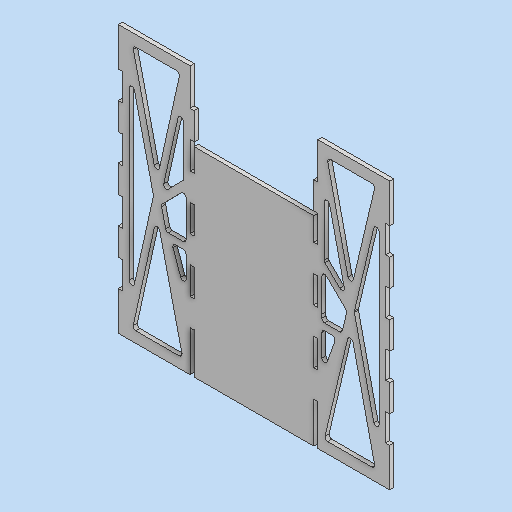
# Autodesk Inventor part: back plate
Saved by Autodesk Inventor 2026 (Build 300175000, 175)
## iProperties
Created: 2026-02-11
Part Number: back plate
Material: Generic
Document SubType Name: Modeling
Designer: mones
Density: 1 g/cm^3
Appearance: Default
Author: mones
Autodesk Inventor part; units mm, degrees
ref_plane "YZ Plane" through (0, 0, 0) normal (1, 0, 0) x (0, 1, 0)
ref_plane "XZ Plane" through (0, 0, 0) normal (0, 1, 0) x (-1, 0, 0)
ref_plane "XY Plane" through (0, 0, 0) normal (0, 0, 1) x (1, 0, 0)
sketch "Sketch1" plane through (0, 0, 0) normal (0, 0, 1) x (1, 0, 0)
  line L0 (-100, 98.5) -> (100, -98.5) construction
  line L1 (100, 98.5) -> (-100, -98.5) construction
  line L2 (-100, 98.5) -> (-100, 70)
  line L3 (-100, 50) -> (-100, 30)
  line L4 (-100, 10) -> (-100, -10)
  line L5 (-100, -30) -> (-100, -50)
  line L6 (-100, -70) -> (-100, -98.5)
  line L7 (-100, 98.5) -> (-100, 95.5)
  line L8 (-100, 98.5) -> (-100, 95.5)
  line L9 (-100, 98.5) -> (-97, 98.5)
  line L10 (-100, -70) -> (-97, -70)
  line L11 (-100, -50) -> (-97, -50)
  line L12 (-100, -30) -> (-97, -30)
  line L13 (-100, -10) -> (-97, -10)
  line L14 (-100, 10) -> (-97, 10)
  line L15 (-100, 30) -> (-97, 30)
  line L16 (-100, 50) -> (-97, 50)
  line L17 (-100, 70) -> (-97, 70)
  line L18 (-100, -98.5) -> (-100, -70)
  line L19 (-100, -50) -> (-100, -30)
  line L20 (-100, -10) -> (-100, 10)
  line L21 (-100, 30) -> (-100, 50)
  line L22 (-100, 70) -> (-100, 98.5)
  line L23 (100, 98.5) -> (97, 98.5)
  line L24 (100, -98.5) -> (100, -70)
  line L25 (100, -50) -> (100, -30)
  line L26 (100, -10) -> (100, 10)
  line L27 (100, 30) -> (100, 50)
  line L28 (100, 70) -> (97, 70)
  line L29 (100, 50) -> (97, 50)
  line L30 (100, 30) -> (97, 30)
  line L31 (100, 10) -> (97, 10)
  line L32 (100, -10) -> (97, -10)
  line L33 (100, -30) -> (97, -30)
  line L34 (100, -50) -> (97, -50)
  line L35 (100, -70) -> (97, -70)
  line L36 (100, -70) -> (100, -98.5)
  line L37 (100, -30) -> (100, -50)
  line L38 (100, 10) -> (100, -10)
  line L39 (100, 98.5) -> (100, 70)
  line L40 (100, 50) -> (100, 30)
  line L41 (-97, -98.5) -> (-47, -98.5)
  line L42 (-47, -98.5) -> (-47, -68.5)
  line L43 (-47, -48.5) -> (-47, -28.5)
  line L44 (-47, -8.5) -> (-47, 11.5)
  line L45 (-47, 31.5) -> (-47, 51.5)
  line L46 (-47, 71.5) -> (-47, 98.5)
  line L47 (-47, 71.5) -> (-44, 71.5)
  line L48 (-47, 51.5) -> (-44, 51.5)
  line L49 (-47, 31.5) -> (-44, 31.5)
  line L50 (-47, 11.5) -> (-44, 11.5)
  line L51 (-47, -8.5) -> (-44, -8.5)
  line L52 (-47, -28.5) -> (-44, -28.5)
  line L53 (-47, -68.5) -> (-44, -68.5)
  line L54 (-47, -98.5) -> (-100, -98.5)
  line L55 (-44, -28.5) -> (-44, -48.5)
  line L56 (-44, -48.5) -> (-47, -48.5)
  line L57 (-44, -98.5) -> (-44, -68.5)
  line L58 (-47, -68.5) -> (-47, -98.5)
  line L59 (-44, -48.5) -> (-44, -28.5)
  line L60 (-47, -28.5) -> (-47, -48.5)
  line L61 (-44, -8.5) -> (-44, 11.5)
  line L62 (-47, 11.5) -> (-47, -8.5)
  line L63 (-44, 31.5) -> (-44, 48.5)
  line L64 (-47, 98.5) -> (-47, 71.5)
  line L65 (-47, 51.5) -> (-47, 31.5)
  line L66 (-100, 98.5) -> (-47, 98.5)
  line L67 (100, -98.5) -> (47, -98.5)
  line L68 (47, -98.5) -> (47, -68.5)
  line L69 (47, -48.5) -> (47, -28.5)
  line L70 (47, -8.5) -> (47, 11.5)
  line L71 (47, 31.5) -> (47, 51.5)
  line L72 (47, 71.5) -> (47, 98.5)
  line L73 (47, 71.5) -> (44, 71.5)
  line L74 (47, 51.5) -> (44, 51.5)
  line L75 (47, 31.5) -> (44, 31.5)
  line L76 (47, 11.5) -> (44, 11.5)
  line L77 (47, -8.5) -> (44, -8.5)
  line L78 (47, -28.5) -> (44, -28.5)
  line L79 (47, -68.5) -> (44, -68.5)
  line L80 (44, -28.5) -> (44, -48.5)
  line L81 (44, -48.5) -> (47, -48.5)
  line L82 (44, -98.5) -> (44, -68.5)
  line L83 (47, -68.5) -> (47, -98.5)
  line L84 (44, -48.5) -> (44, -28.5)
  line L85 (47, -28.5) -> (47, -48.5)
  line L86 (44, -8.5) -> (44, 11.5)
  line L87 (47, 11.5) -> (47, -8.5)
  line L88 (44, 31.5) -> (44, 48.5)
  line L89 (47, 98.5) -> (47, 71.5)
  line L90 (47, 51.5) -> (47, 31.5)
  line L91 (100, -98.5) -> (47, -98.5)
  line L92 (44, -98.5) -> (-44, -98.5)
  line L93 (47, 98.5) -> (97, 98.5)
  line L94 (47, 98.5) -> (100, 98.5)
  line L95 (-97, 98.5) -> (-47, 98.5)
  line L96 (-97, 70) -> (-97, 50)
  line L97 (-97, 30) -> (-97, 10)
  line L98 (-97, -10) -> (-97, -30)
  line L99 (-97, -50) -> (-97, -70)
  line L100 (97, -50) -> (97, -70)
  line L101 (97, -10) -> (97, -30)
  line L102 (97, 30) -> (97, 10)
  line L103 (97, 70) -> (97, 50)
  line L104 (44, 71.5) -> (44, 51.5)
  line L105 (44, 48.5) -> (-44, 48.5)
  line L106 (-44, 71.5) -> (-44, 51.5)
  point P0 (0, 0)
  constraints: 214 end point, 100 perpendicular, 37 parallel, 7 collinear, 4 point on line, 3 horizontal, 2 midpoint
extrude "Extrusion1" add sketch "Sketch1" along normal blind 3
sketch "Sketch2" plane through (0, 0, 3) normal (0, 0, 1) x (1, 0, 0)
  line L0 (-100, -70) -> (-100, -98.5) projected
  line L1 (-100, -98.5) -> (-47, -98.5) projected
  line L2 (-47, -98.5) -> (-47, -68.5) projected
  line L3 (-47, -68.5) -> (-44, -68.5) projected
  line L4 (-44, -68.5) -> (-44, -98.5) projected
  line L5 (-44, -98.5) -> (44, -98.5) projected
  line L6 (44, -98.5) -> (44, -68.5) projected
  line L7 (44, -68.5) -> (47, -68.5) projected
  line L8 (47, -68.5) -> (47, -98.5) projected
  line L9 (47, -98.5) -> (100, -98.5) projected
  line L10 (100, -98.5) -> (100, -70) projected
  line L11 (100, -70) -> (97, -70) projected
  line L12 (97, -70) -> (97, -50) projected
  line L13 (97, -50) -> (100, -50) projected
  line L14 (100, -50) -> (100, -30) projected
  line L15 (100, -30) -> (97, -30) projected
  line L16 (97, -30) -> (97, -10) projected
  line L17 (97, -10) -> (100, -10) projected
  line L18 (100, -10) -> (100, 10) projected
  line L19 (100, 10) -> (97, 10) projected
  line L20 (97, 10) -> (97, 30) projected
  line L21 (97, 30) -> (100, 30) projected
  line L22 (100, 30) -> (100, 50) projected
  line L23 (100, 50) -> (97, 50) projected
  line L24 (97, 50) -> (97, 70) projected
  line L25 (97, 70) -> (100, 70) projected
  line L26 (100, 70) -> (100, 98.5) projected
  line L27 (100, 98.5) -> (47, 98.5) projected
  line L28 (47, 98.5) -> (47, 71.5) projected
  line L29 (47, 71.5) -> (44, 71.5) projected
  line L30 (44, 71.5) -> (44, 51.5) projected
  line L31 (44, 51.5) -> (47, 51.5) projected
  line L32 (47, 51.5) -> (47, 31.5) projected
  line L33 (47, 31.5) -> (44, 31.5) projected
  line L34 (44, 31.5) -> (44, 48.5) projected
  line L35 (44, 48.5) -> (-44, 48.5) projected
  line L36 (-44, 48.5) -> (-44, 31.5) projected
  line L37 (-44, 31.5) -> (-47, 31.5) projected
  line L38 (-47, 31.5) -> (-47, 51.5) projected
  line L39 (-47, 51.5) -> (-44, 51.5) projected
  line L40 (-44, 51.5) -> (-44, 71.5) projected
  line L41 (-44, 71.5) -> (-47, 71.5) projected
  line L42 (-47, 71.5) -> (-47, 98.5) projected
  line L43 (-47, 98.5) -> (-100, 98.5) projected
  line L44 (-100, 98.5) -> (-100, 70) projected
  line L45 (-100, 70) -> (-97, 70) projected
  line L46 (-97, 70) -> (-97, 50) projected
  line L47 (-97, 50) -> (-100, 50) projected
  line L48 (-100, 50) -> (-100, 30) projected
  line L49 (-100, 30) -> (-97, 30) projected
  line L50 (-97, 30) -> (-97, 10) projected
  line L51 (-97, 10) -> (-100, 10) projected
  line L52 (-100, 10) -> (-100, -10) projected
  line L53 (-100, -10) -> (-97, -10) projected
  line L54 (-97, -10) -> (-97, -30) projected
  line L55 (-97, -30) -> (-100, -30) projected
  line L56 (-100, -30) -> (-100, -50) projected
  line L57 (-100, -50) -> (-97, -50) projected
  line L58 (-97, -50) -> (-97, -70) projected
  line L59 (-97, -70) -> (-100, -70) projected
  line L60 (-47, 11.5) -> (-44, 11.5) projected
  line L61 (-44, 11.5) -> (-44, -8.5) projected
  line L62 (-44, -8.5) -> (-47, -8.5) projected
  line L63 (-47, -8.5) -> (-47, 11.5) projected
  line L64 (47, -8.5) -> (44, -8.5) projected
  line L65 (44, -8.5) -> (44, 11.5) projected
  line L66 (44, 11.5) -> (47, 11.5) projected
  line L67 (47, 11.5) -> (47, -8.5) projected
  line L68 (44, -28.5) -> (47, -28.5) projected
  line L69 (47, -28.5) -> (47, -48.5) projected
  line L70 (47, -48.5) -> (44, -48.5) projected
  line L71 (44, -48.5) -> (44, -28.5) projected
  line L72 (-47, -28.5) -> (-44, -28.5) projected
  line L73 (-44, -28.5) -> (-44, -48.5) projected
  line L74 (-44, -48.5) -> (-47, -48.5) projected
  line L75 (-47, -48.5) -> (-47, -28.5) projected
  line L76 (51.6706, 24.0323) -> (51.7144, 61.2135)
  line L77 (50.0544, 13.1843) -> (49.999, -11.4223)
  line L78 (50, -39.3414) -> (50, -23)
  line L79 (-50.0184, -23.0136) -> (-50.0321, -39.1948)
  line L80 (-50, 13.0588) -> (-50, -11.5)
  line L81 (47, 31.5) -> (44, 31.5)
  line L82 (-47, 90.5) -> (-46.8853, 90.4938)
  line L83 (86.8574, 90.5429) -> (56.2449, 90.5429)
  line L84 (-56.9156, 90.4938) -> (-86.863, 90.4938)
  line L85 (-100, 98.5) -> (-52, 98.5)
  line L86 (52, 98.5) -> (97, 98.5)
  line L87 (60.4802, 84.2685) -> (35.0176, 85.6502)
  line L88 (100, 98.5) -> (100, 70)
  line L89 (100, -30) -> (100, -50)
  line L90 (54.2742, -90.4539) -> (86.9163, -90.4539)
  line L91 (47, -98.5) -> (44, -98.5)
  line L92 (-44, -98.5) -> (-100, -98.5)
  line L93 (-86.9859, -90.4916) -> (-54.9903, -90.4916)
  line L94 (-100, -98.5) -> (-100, -70)
  line L95 (-100, -50) -> (-100, -30)
  line L96 (-100, -10) -> (-100, 10)
  line L97 (-100, 30) -> (-100, 98.5)
  line L98 (-51.9599, 60.5849) -> (-52, 26.5)
  line L99 (-95.4597, 94.3495) -> (-47.5647, -89.9349) construction
  line L100 (-52.3399, -91.0567) -> (-90.4937, 95.4882) construction
  line L101 (-93.4655, -85.5459) -> (-49.5589, 89.9605) construction
  line L102 (-54.9518, 88.1154) -> (-88.6187, -86.617) construction
  line L103 (88.5429, -86.5805) -> (54.3944, 91.0824) construction
  line L104 (49.5589, 89.9605) -> (93.4655, -85.5459) construction
  line L105 (48.5891, -85.5203) -> (94.4353, 89.9349) construction
  line L106 (89.4893, 90.9575) -> (52.6562, -86.6086) construction
  line L107 (54.2942, 88.1013) -> (69.2477, 22.0411)
  line L108 (73.9725, 1.696) -> (88.2518, -61.386)
  line L109 (73.1444, 22.0213) -> (88.8035, 88.0816)
  line L110 (88.2563, 62.8381) -> (73.977, 2.5988)
  line L111 (66.5133, 13.728) -> (55.665, 61.6527)
  line L112 (69.0254, -17.5526) -> (52.6562, -86.6086)
  line L113 (88.867, -88.0123) -> (72.9221, -17.5723)
  line L114 (52.6562, -86.6086) -> (52.3281, -87.9926)
  line L115 (92.2024, -60.9445) -> (92.2024, 62.3768)
  line L116 (-73.4539, 22.0984) -> (-88.8109, 88.0401)
  line L117 (-69.5535, 22.1188) -> (-55.2275, 86.6843)
  line L118 (-88.0475, -61.101) -> (-74.1053, 1.7347)
  line L119 (-73.3278, -17.7028) -> (-88.9385, -88.0583)
  line L120 (-88.0521, 62.4881) -> (-74.1099, 2.6215)
  line L121 (-69.4274, -17.6824) -> (-53.0424, -88.0379)
  line L122 (-92, 62.0345) -> (-92, -60.6678)
  line L123 (47.643, -57.6667) -> (66.4978, -19.3333) construction
  line L124 (61.7837, -17.6667) -> (52.357, -59.3333) construction
  line L125 (51.999, -16) -> (63.152, -16)
  line L126 (49.999, -16) -> (64.1404, -20.9995) construction
  line L127 (64.1408, -16) -> (50, -21) construction
  line L128 (52.2661, 22.606) -> (63.1582, 11.8625)
  line L129 (67.6753, 0.5811) -> (53.4589, 14.6037)
  line L130 (52.5563, 22.3198) -> (67.4137, 0.8392) construction
  line L131 (70.8742, 4.3439) -> (49.1242, 18.7741) construction
  line L132 (64.1408, -16) -> (64.7334, -16)
  line L133 (52.5563, 22.3198) -> (52.2661, 22.606)
  line L134 (59.9992, 11.559) -> (60.059, 11.5)
  line L135 (65.0981, -14.4613) -> (68.2169, -1.3041)
  line L136 (53.8856, -40.008) -> (59.6626, -23.6666)
  line L137 (49.999, -11.4223) -> (49.999, -14)
  line L138 (50, -23) -> (50, -25.5)
  line L139 (57.777, -21) -> (52, -21)
  line L140 (-63.1153, -16.0025) -> (-52.0017, -16.0119)
  line L141 (-64.1172, -16.0017) -> (-50.0167, -21.0136) construction
  line L142 (-50, -16.0136) -> (-64.1069, -21.0076) construction
  line L143 (-63.0471, 11.7994) -> (-52.7838, 22.2516)
  line L144 (-53.427, 14.4601) -> (-67.5042, 0.1238)
  line L145 (-70.7327, 3.9724) -> (-49.2162, 18.7484) construction
  line L146 (-52.7838, 22.2516) -> (-67.1651, 0.4692) construction
  line L147 (-66.4619, -19.3356) -> (-47.574, -57.6528) construction
  line L148 (-52.2866, -59.3234) -> (-61.7492, -17.665) construction
  line L149 (-52.7838, 22.2516) -> (-52.2215, 22.8243)
  line L150 (-67.1651, 0.4692) -> (-67.5042, 0.1238)
  line L151 (-52.0167, -21.0119) -> (-57.7528, -21.0071)
  line L152 (-53.9177, -39.8598) -> (-59.6401, -23.6737)
  line L153 (-65.0615, -14.4562) -> (-68.025, -1.731)
  line L154 (-50, -11.5) -> (-50, -14.0119)
  line L155 (-50.0184, -23.0136) -> (-50.0205, -25.5136)
  line L156 (-51.6757, 24.5543) -> (-52, 26.5)
  line L157 (-55.9124, 61.0205) -> (-66.4267, 13.6339)
  line L158 (-41, -51.5) -> (-41, -51.4556)
  line L159 (-49.9765, 26.4877) -> (-49.978, 26.5013)
  arc A0 (-86.863, 90.4938) -> (-88.8109, 88.0401) centre (-86.863, 88.4938) ccw
  arc A1 (-54.9518, 88.1154) -> (-56.9156, 90.4938) centre (-56.9156, 88.4938) ccw
  arc A2 (-73.4539, 22.0984) -> (-69.5535, 22.1188) centre (-71.506, 22.552) ccw
  arc A3 (-51.9599, 60.5849) -> (-55.9124, 61.0205) centre (-53.9599, 60.5873) ccw
  arc A4 (-66.4267, 13.6339) -> (-63.0471, 11.7994) centre (-64.4741, 13.2007) ccw
  arc A5 (-52.2215, 22.8243) -> (-51.6757, 24.5543) centre (-53.6485, 24.2255) ccw
  arc A6 (-50, 13.0588) -> (-53.427, 14.4601) centre (-52, 13.0588) ccw
  arc A7 (-52.0017, -16.0119) -> (-50, -14.0119) centre (-52, -14.0119) ccw
  arc A8 (-65.0615, -14.4562) -> (-63.1153, -16.0025) centre (-63.1136, -14.0025) ccw
  arc A9 (-67.5042, 0.1238) -> (-68.025, -1.731) centre (-66.0772, -1.2774) ccw
  arc A10 (-74.1053, 1.7347) -> (-74.1099, 2.6215) centre (-76.0578, 2.1679) ccw
  arc A11 (-88.0521, 62.4881) -> (-92, 62.0345) centre (-90, 62.0345) ccw
  arc A12 (-92, -60.6678) -> (-88.0475, -61.101) centre (-90, -60.6678) ccw
  arc A13 (-88.9385, -88.0583) -> (-86.9859, -90.4916) centre (-86.9859, -88.4916) ccw
  arc A14 (-54.9903, -90.4916) -> (-53.0424, -88.0379) centre (-54.9903, -88.4916) ccw
  arc A15 (-69.4274, -17.6824) -> (-73.3278, -17.7028) centre (-71.3752, -18.136) ccw
  arc A16 (-57.7528, -21.0071) -> (-59.6401, -23.6737) centre (-57.7545, -23.0071) ccw
  arc A17 (-50.0184, -23.0136) -> (-52.0167, -21.0119) centre (-52.0184, -23.0119) ccw
  arc A18 (-53.9177, -39.8598) -> (-50.0321, -39.1948) centre (-52.0321, -39.1931) ccw
  line L160 (-54.9518, 88.1154) -> (-55.2702, 86.4916)
  arc A19 (55.665, 61.6527) -> (51.7144, 61.2135) centre (53.7144, 61.2111) ccw
  arc A20 (51.6706, 24.0323) -> (52.2661, 22.606) centre (53.6706, 24.0299) ccw
  arc A21 (53.4589, 14.6037) -> (50.0544, 13.1843) centre (52.0544, 13.1798) ccw
  arc A22 (63.1582, 11.8625) -> (66.5133, 13.728) centre (64.5627, 13.2864) ccw
  arc A23 (69.2477, 22.0411) -> (73.1444, 22.0213) centre (71.1983, 22.4826) ccw
  arc A24 (56.2449, 90.5429) -> (54.2942, 88.1013) centre (56.2449, 88.5429) ccw
  arc A25 (88.8035, 88.0816) -> (86.8574, 90.5429) centre (86.8574, 88.5429) ccw
  arc A26 (92.2024, 62.3768) -> (88.2563, 62.8381) centre (90.2024, 62.3768) ccw
  arc A27 (73.977, 2.5988) -> (73.9725, 1.696) centre (75.9231, 2.1375) ccw
  arc A28 (88.2518, -61.386) -> (92.2024, -60.9445) centre (90.2024, -60.9445) ccw
  arc A29 (86.9163, -90.4539) -> (88.867, -88.0123) centre (86.9163, -88.4539) ccw
  arc A30 (52.3281, -87.9926) -> (54.2742, -90.4539) centre (54.2742, -88.4539) ccw
  arc A31 (59.6626, -23.6666) -> (57.777, -21) centre (57.777, -23) ccw
  arc A32 (52, -21) -> (50, -23) centre (52, -23) ccw
  arc A33 (72.9221, -17.5723) -> (69.0254, -17.5526) centre (70.9715, -18.0139) ccw
  arc A34 (49.999, -14) -> (51.999, -16) centre (51.999, -14) ccw
  arc A35 (63.152, -16) -> (65.0981, -14.4613) centre (63.152, -14) ccw
  arc A36 (68.2169, -1.3041) -> (67.6753, 0.5811) centre (66.2709, -0.8428) ccw
  arc A37 (50, -39.3414) -> (53.8856, -40.008) centre (52, -39.3414) ccw
  point P0 (-52.4555, -90.4916)
  point P1 (89.4033, 90.5429)
  point P2 (57.0704, -18.5)
  point P3 (-51.5084, 23.5504)
  dimension "d55" = 2
  dimension "d56" = 2
  dimension "d57" = 2
  dimension "d58" = 2
  dimension "d59" = 2
  dimension "d60" = 2
  dimension "d61" = 2
  dimension "d62" = 2
  dimension "d63" = 2
  dimension "d64" = 2
  dimension "d65" = 2
  dimension "d66" = 2
  dimension "d67" = 2
  dimension "d68" = 2
  dimension "d69" = 2
  constraints: 182 end point, 76 point on circle, 76 tangent, 41 parallel, 39 point on line, 38 centre point, 23 equal radius, 6 perpendicular, 2 horizontal, 2 midpoint, 2 vertical
  measures "d55" radius of A0
  measures "d56" radius of A6
  measures "d57" radius of A7
  measures "d58" radius of A9
  measures "d59" radius of A10
  measures "d60" radius of A14
  measures "d61" radius of A18
  measures "d62" radius of A19
  measures "d63" radius of A21
  measures "d64" radius of A22
  measures "d65" radius of A24
  measures "d66" radius of A25
  measures "d67" radius of A30
  measures "d68" radius of A33
  measures "d69" radius of A37
extrude "Extrusion2" cut sketch "Sketch2" against normal blind 3 contours L76 A19 L111 A22 L128 A20 | A21 L129 A36 L135 A35 L125 A34 L137 L77 | L78 A32 L139 A31 L136 A37 | L79 A18 L152 A16 L151 A17 | L80 L154 A7 L140 A8 L153 A9 L144 A6 | A25 L109 A23 L107 A24 L83 | A1 L160 L117 A2 L116 A0 L84 | A30 L114 L112 A33 L113 A29 L90 | A13 L119 A15 L121 A14 L93 | L98 L156 A5 L149 L143 A4 L157 A3 | A27 L110 A26 L115 A28 L108 | A12 L122 A11 L120 A10 L118
body "Solid1"
